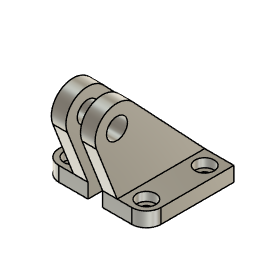
middle_pulley_mount v3 (Autodesk Fusion 360 design; units mm, degrees)
Autodesk Fusion 360 part; units mm, degrees
note: some values were not read from the file. Set by a fixed rule: which sketch regions a step uses.
sketch "Sketch1" plane through (0, 0, 0) normal (0, 0, 1) x (1, 0, 0)
  line L0 (0, 0) -> (15, 0)
  line L1 (15, 0) -> (15, 30)
  line L2 (15, 30) -> (0, 30)
  line L3 (0, 30) -> (0, 0)
  circle A0 centre (10, 25) radius 1.6
  circle A1 centre (10, 5) radius 1.6
  dimension "d1" = 15
  dimension "d2" = 30
  dimension "d3" = 3.2
  dimension "d4" = 3.2
  dimension "d5" = 5
  dimension "d7" = 5
  constraint horizontal L0
  constraint vertical L1
  constraint horizontal L2
  constraint vertical L3
  constraint coincident L0.start L3.end
  measures "d1" distance of L1 L3
  measures "d2" distance of L0.start L2.end
  measures "d3" diameter of A0
  measures "d4" diameter of A1
  measures "d5" distance of L2 A0.centre
  measures "d7" distance of L0 A1.centre
extrude "Extrude1" add sketch "Sketch1" along normal blind 5 makes body 1
sketch "Sketch2" plane through (0, 0, 0) normal (-1, 0, 0) x (0, -1, 0)
  line L0 (-30, 0) -> (0, 0)
  line L1 (0, 0) -> (0, 5)
  line L2 (0, 5) -> (-30, 5)
  line L3 (-30, 5) -> (-30, 0)
  circle A0 centre (0.0771, 26) radius 3.6
  circle A1 centre (0.0771, 26) radius 7.5
  line L4 (0, 5) -> (7.0726, 23.2958)
  line L5 (-30, 5) -> (-5.3831, 31.1417)
  dimension "d10" = 7.2
  dimension "d11" = 15
  dimension "d16" = 26
  constraint concentric A0 A1
  constraint coincident L1.end L2.start
  constraint coincident A1 L4.end
  constraint tangent A1 L4
  constraint coincident L2.end L3.start
  constraint coincident A1 L5.end
  constraint tangent A1 L5
  measures "d10" diameter of A0
  measures "d11" diameter of A1
  measures "d16" distance of L0 A0.centre
extrude "Extrude2" add sketch "Sketch2" against normal blind 5 contours L2 A1 L4 L5 | A1 bodies 1
sketch "Sketch3" plane through (0, 0, 5) normal (0, 0, 1) x (-1, 0, 0)
  line L0 (-5, -30) -> (-5, 0)
  line L1 (-5, 0) -> (-15, 0)
  line L2 (-15, 0) -> (-15, -30)
  line L3 (-15, -30) -> (-5, -30)
  circle A0 centre (-10, -25) radius 1.6
  circle A1 centre (-10, -5) radius 1.6
  circle A2 centre (-10, -5) radius 3.25
  circle A3 centre (-10, -25) radius 3.25
  dimension "d17" = 6.5
  dimension "d18" = 6.5
  constraint concentric A1 A2
  constraint concentric A0 A3
  measures "d17" diameter of A2
  measures "d18" diameter of A3
extrude "Extrude3" cut sketch "Sketch3" against normal blind 3 contours A2 | A3 bodies 1
mirror "Mirror2" about plane through (0, 0, 0) normal (1, 0, 0) of bodies 1 makes body 2
move_body "Move2" bodies 2 to x (1, 0, 0) y (0, 1, 0) z (0, 0, 1) at (-5, 0, 0)
fillet "Fillet1" radius 5 2 edges at (15, 0, 2.5) (-20, 0, 2.5) on bodies 1 2
